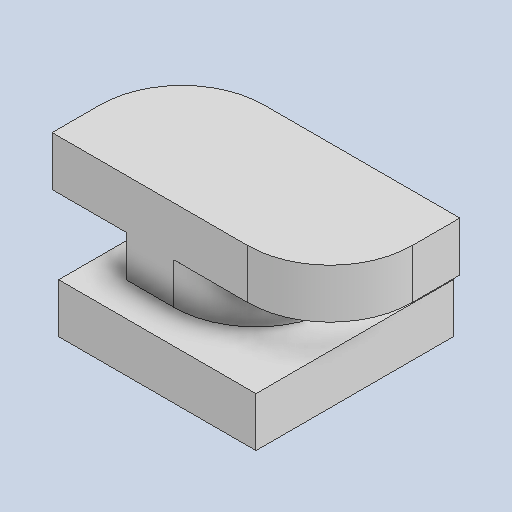
# Autodesk Inventor part: test
Saved by Autodesk Inventor 2025 (Build 290162000, 162)
## iProperties
Created: 2025-07-09
Part Number: test
Material: Generic
Document SubType Name: Modeling
Designer: Pravoslav
Density: 1 g/cm^3
Appearance: Default
Author: Pravoslav
Autodesk Inventor part; units mm, degrees
ref_plane "YZ Plane" through (0, 0, 0) normal (1, 0, 0) x (0, 1, 0)
ref_plane "XZ Plane" through (0, 0, 0) normal (0, 1, 0) x (-1, 0, 0)
ref_plane "XY Plane" through (0, 0, 0) normal (0, 0, 1) x (1, 0, 0)
sketch "Sketch1" plane through (0, 0, 0) normal (0, 1, 0) x (-1, 0, 0)
  line L0 (3.95, 3.95) -> (-3.95, 3.95)
  line L1 (-3.95, 3.95) -> (-3.95, -3.95)
  line L2 (-3.95, -3.95) -> (3.95, -3.95)
  line L3 (3.95, -3.95) -> (3.95, 3.95)
  line L4 (3.95, 3.95) -> (-3.95, -3.95) construction
  line L5 (-3.95, 3.95) -> (3.95, -3.95) construction
  point P0 (0, 0)
  dimension "d0" = 7.9
  dimension "d1" = 7.9
  constraints: 12 end point, 2 midpoint, 2 parallel, 1 horizontal, 1 perpendicular
  measures "d0" distance of L2.end L1.end
  measures "d1" distance of L1.end L0.end
extrude "Extrusion1" add sketch "Sketch1" along normal blind 2.5
sketch "Sketch2" plane through (0, 2.5, 0) normal (0, 1, 0) x (1, 0, 0)
  line L0 (-8.45, -3.95) -> (8.45, -3.95)
  line L1 (8.45, -3.95) -> (8.45, 3.95)
  line L2 (8.45, 3.95) -> (-8.45, 3.95)
  line L3 (-8.45, 3.95) -> (-8.45, -3.95)
  line L4 (-8.45, -3.95) -> (8.45, 3.95) construction
  line L5 (8.45, -3.95) -> (-8.45, 3.95) construction
  point P0 (0, 0)
  dimension "d4" = 16.9
  dimension "d5" = 7.9
  constraints: 12 end point, 2 midpoint, 2 parallel, 1 horizontal, 1 perpendicular
  measures "d4" distance of L2.end L1.end
  measures "d5" distance of L1.end L0.end
extrude "Extrusion2" add sketch "Sketch2" along normal blind 3
sketch "Sketch3" plane through (0, 0, 0) normal (0, -1, 0) x (1, 0, 0)
  line L0 (-6, -6) -> (6, -6)
  line L1 (6, -6) -> (6, 6)
  line L2 (6, 6) -> (-6, 6)
  line L3 (-6, 6) -> (-6, -6)
  line L4 (-6, -6) -> (6, 6) construction
  line L5 (6, -6) -> (-6, 6) construction
  point P0 (0, 0)
  dimension "d8" = 12
  dimension "d9" = 12
  constraints: 12 end point, 2 midpoint, 2 parallel, 1 horizontal, 1 perpendicular
  measures "d8" distance of L2.end L1.end
  measures "d9" distance of L1.end L0.end
extrude "Extrusion3" add sketch "Sketch3" along normal blind 3
fillet "Fillet1" radius 5 4 edges at (-3.95, 1.25, -3.95) (-8.45, 4, -3.95) (8.45, 4, 3.95) (3.95, 1.25, 3.95)
body "Solid1"
